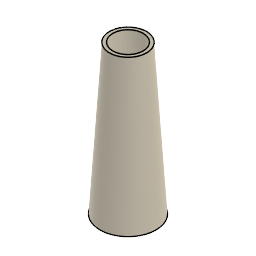
compressor_to_chamber_connection_v0 (Autodesk Fusion 360 design; units mm, degrees)
part number: 2026-09-02-21-26-19-197
Autodesk Fusion 360 part; units mm, degrees
sketch "Sketch1" plane through (0, 0, 0) normal (0, 0, 1) x (1, 0, 0)
  circle A0 centre (0, 0) radius 37.75
  dimension "d5" = 75.5
  constraint coincident A0.centre origin
  measures "d5" diameter of A0
ref_plane "WorkPlane1" through (0, 0, 200) normal (0, 0, 1) x (1, 0, 0)
sketch "Sketch2" plane through (0, 0, 200) normal (0, 0, 1) x (1, 0, 0)
  circle A0 centre (0, 0) radius 25
  dimension "d8" = 50
  constraint coincident A0.centre origin
  measures "d8" diameter of A0
loft "Loft1" add profiles "Sketch1", "Sketch2" section 1 section 2
shell "Shell1" thickness 4.5 removed faces 2 at (-6.7759, -1.242, 200) at (9.2242, 8.5588, 0)
equation "hose_end1_ID = 75.5 mm" comment "compressor lip, confirmed"
equation "hose_end2_ID = 50 mm" comment "placeholder, not confirmed"
equation "hose_length = 200 mm"
equation "wall_thickness = 4.5 mm"
equation "d5 = hose_end1_ID"
equation "d6 = hose_length"
equation "d8 = hose_end2_ID"
equation "d9 = wall_thickness"
